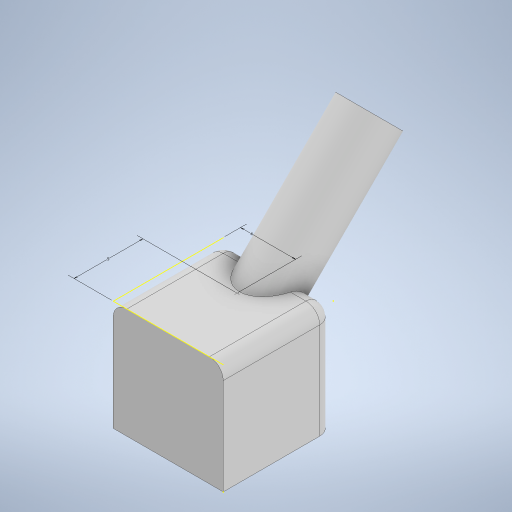
# Autodesk Inventor part: as2
Saved by Autodesk Inventor 2023 (Build 270158000, 158)
## iProperties
Created: 2022-12-05
Part Number: as2
Material: Generic
Document SubType Name: Modeling
Designer: daarn
Density: 1 g/cm^3
Appearance: Default
Author: daarn
Autodesk Inventor part; units mm, degrees
ref_plane "YZ Plane" through (0, 0, 0) normal (1, 0, 0) x (0, 1, 0)
ref_plane "XZ Plane" through (0, 0, 0) normal (0, 1, 0) x (-1, 0, 0)
sketch "Sketch1" plane through (0, 0, 0) normal (0, 0, 1) x (1, 0, 0)
  line L0 (-8, 8) -> (0, 8)
  line L1 (0, 8) -> (0, 0)
  line L2 (0, 0) -> (-8, 0)
  line L3 (-8, 0) -> (-8, 8)
  dimension "d0" = 8
  dimension "d1" = 8
  constraints: 8 end point, 2 parallel, 1 coincident, 1 horizontal, 1 perpendicular
  measures "d0" distance of L1.end L2.end
  measures "d1" distance of L0.end L1.end
extrude "Extrusion1" add sketch "Sketch1" along normal blind 8
sketch "Sketch5" plane through (0, 0, 8) normal (0, 0, 1) x (1, 0, 0)
  point P0 (0, 0)
sketch "Sketch8" plane through (-8, 8, 0) normal (0, 1, 0) x (1, 0, 0)
  line L0 (8, -8) -> (0, -8) projected
  line L1 (0, 0) -> (0, -8) projected
  point P0 (8, 0)
  point P1 (4, -3)
  dimension "d14" = 5
  dimension "d15" = 4
  measures "d14" distance from line of L0 point (4, -3)
  measures "d15" distance from line of L1 point (4, -3)
ref_plane "Work Plane3" through (0, 8, 8) normal (0, -0.7071068, 0.7071068) x (-1, 0, 0)
sketch "Sketch11" plane through (0, 8, 8) normal (0, -0.7071068, 0.7071068) x (-1, 0, 0)
  line L0 (8, 5.6569) -> (0, 5.6569) projected
  circle A0 centre (4, 5.6569) radius 2
  point P0 (0, 11.3137)
  dimension "d21" = 4
  constraints: 1 centre point, 1 midpoint
  measures "d21" diameter of A0
extrude "Extrusion4" add sketch "Sketch11" against normal blind 15
sketch "Sketch12" plane through (-8, 0, 0) normal (0, -1, 0) x (1, 0, 0)
  point P0 (8, 0)
  point P1 (4, 4)
  dimension "d24" = 4
  dimension "d25" = 4
  measures "d24" horizontal distance of point (8, 0) point (4, 4)
  measures "d25" horizontal distance of point (4, 4) point (8, 0)
hole "Hole1" at (-4, 0, 4) direction (0, 1, 0) diameter 3.242 depth 5 tip angle 118 thread size "M4x0.7" class "6H" standard "ISO Metric profile"
fillet "Fillet1" radius 1 6 edges at (-7, 8, 0) (-8, 8, 4) (-8, 4, 0) (-1, 8, 0) (0, 8, 4) (0, 4, 0)
body "Solid1"
